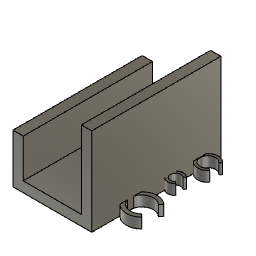
3dprentun v2 (Autodesk Fusion 360 design; units mm, degrees)
Autodesk Fusion 360 part; units mm, degrees
sketch "Sketch1" plane through (0, 0, 0) normal (0, 0, 1) x (1, 0, 0)
  line L0 (0, 0) -> (30.5, 0)
  line L1 (30.5, 0) -> (30.5, 50)
  line L2 (30.5, 50) -> (0, 50)
  line L3 (0, 50) -> (0, 0)
  dimension "d3" = 30.5
  dimension "d5" = 50
  constraint coincident L0.start L3.end
  constraint horizontal L0
  constraint perpendicular L0 L1
  constraint perpendicular L1 L2
  constraint perpendicular L0 L3
  measures "d3" distance of L0.start L0.end
  measures "d5" distance of L0.end L1.end
extrude "Extrude1" add sketch "Sketch1" along normal blind 19 makes body 1
sketch "Sketch2" plane through (0, 0, 19) normal (0, 0, 1) x (-1, 0, 0)
  line L0 (0, -50) -> (0, 0)
  line L1 (0, 0) -> (-30.5, 0)
  line L2 (-30.5, 0) -> (-30.5, -50)
  line L3 (-30.5, -50) -> (0, -50)
  line L4 (0, -50) -> (-4, -50)
  line L5 (-4, -50) -> (-26.5, -50)
  line L6 (-26.5, -50) -> (-26.5, 0)
  line L7 (-26.5, 0) -> (-4, 0)
  line L8 (-4, 0) -> (-4, -50)
  dimension "d9" = 4
  dimension "d10" = 22.5
  constraint coincident L0.start L3.end
  constraint coincident L3 L4.end
  constraint horizontal L5
  constraint vertical L6
  constraint horizontal L7
  constraint vertical L8
  constraint coincident L1 L6.end
  measures "d9" distance of L0.start L4.end
  measures "d10" distance of L6.end L7.end
extrude "Extrude2" cut sketch "Sketch2" against normal blind 15 contours L1 L3 L5 L6 L7 L8 bodies 1
sketch "Sketch3" plane through (0, 0, 4) normal (0, 0, 1) x (-1, 0, 0)
  line L0 (-4, 0) -> (-26.5, 0)
  line L1 (-26.5, 0) -> (-26.5, -50)
  line L2 (-26.5, -50) -> (-4, -50)
  line L3 (-4, -50) -> (-4, 0)
  circle A0 centre (-53.2527, -36.6298) radius 3
  circle A1 centre (-53.2527, -36.6298) radius 4
  dimension "d15" = 6
  dimension "d16" = 8
  constraint concentric A0 A1
  measures "d15" diameter of A0
  measures "d16" diameter of A1
extrude "Extrude3" add sketch "Sketch3" along normal blind 4 separate body contours A1 makes body 2
sketch "Sketch4" plane through (0, 0, 8) normal (0, 0, 1) x (-1, 0, 0)
  circle A0 centre (-53.2527, -36.6298) radius 3
  circle A1 centre (-53.2527, -36.6298) radius 4
  arc A2 (-56.3995, -34.1605) -> (-56.3725, -39.1331) centre (-53.2527, -36.6298) ccw
  line L0 (-56.3995, -34.1605) -> (-53.2527, -36.6298)
  line L1 (-53.2527, -36.6298) -> (-56.3725, -39.1331)
  constraint coincident A1 A2.end
  constraint coincident A0.centre A1.centre
extrude "Extrude4" cut sketch "Sketch4" against normal blind 4 contours A0 A1 A2 L0 L1 bodies 2
move_body "Move1" bodies 2 to x (1, 0, 0) y (0, 1, 0) z (0, 0, 1) at (-19.6373, -0.4364, 0)
move_body "Move2" bodies 2 to x (1, 0, 0) y (0, 1, 0) z (0, 0, 1) at (0, 5.6722, -3.8196)
combine "Combine1" operation add target body 2 tool bodies 1 keep tools
sketch "Sketch5" plane through (0, 0, 4) normal (0, 0, 1) x (-1, 0, 0)
  line L0 (-4, 0) -> (-26.5, 0)
  line L1 (-26.5, 0) -> (-26.5, -50)
  line L2 (-26.5, -50) -> (-4, -50)
  line L3 (-4, -50) -> (-4, 0)
  circle A0 centre (-41, -32) radius 2
  circle A1 centre (-41, -32) radius 3
  dimension "d21" = 4
  dimension "d22" = 6
  constraint concentric A0 A1
  measures "d21" diameter of A0
  measures "d22" diameter of A1
extrude "Extrude5" add sketch "Sketch5" along normal blind 4 separate body contours A1 makes body 3
sketch "Sketch6" plane through (0, 0, 8) normal (0, 0, 1) x (-1, 0, 0)
  circle A0 centre (-41, -32) radius 2
  circle A1 centre (-41, -32) radius 3
  arc A2 (-43.3273, -30.1069) -> (-42.8931, -34.3273) centre (-41, -32) ccw
  line L0 (-41, -32) -> (-43.3273, -30.1069) construction
  line L1 (-41, -32) -> (-42.8931, -34.3273) construction
  line L2 (-41, -32) -> (-42.8931, -34.3273)
  line L3 (-41, -32) -> (-43.3273, -30.1069)
  dimension "d25" = 90
  constraint coincident A1 A2.end
  constraint coincident A0.centre A1.centre
  measures "d25" angle of L0 L1
extrude "Extrude6" cut sketch "Sketch6" against normal blind 4 contours A0 A1 A2 L2 L3 bodies 3
move_body "Move3" bodies 3 to x (0.996195, -0.087156, 0) y (0.087156, 0.996195, 0) z (0, 0, 1) at (-2.633, 3.6952, 0)
move_body "Move4" bodies 3 to x (1, 0, 0) y (0, 1, 0) z (0, 0, 1) at (-8.6186, -1.091, 0)
move_body "Move5" bodies 3 to x (1, 0, 0) y (0, 1, 0) z (0, 0, 1) at (0, -0.3273, -3.9275)
sketch "Sketch7" plane through (0, 0, 4) normal (0, 0, 1) x (-1, 0, 0)
  line L0 (-4, 0) -> (-26.5, 0)
  line L1 (-26.5, 0) -> (-26.5, -50)
  line L2 (-26.5, -50) -> (-4, -50)
  line L3 (-4, -50) -> (-4, 0)
  circle A0 centre (-44, -24) radius 4.5
  circle A1 centre (-44, -24) radius 6
  dimension "d29" = 9
  dimension "d30" = 12
  constraint concentric A0 A1
  measures "d29" diameter of A0
  measures "d30" diameter of A1
extrude "Extrude7" add sketch "Sketch7" along normal blind 4 separate body contours A1 makes body 4
sketch "Sketch8" plane through (0, 0, 8) normal (0, 0, 1) x (-1, 0, 0)
  circle A0 centre (-44, -24) radius 4.5
  circle A1 centre (-44, -24) radius 6
  arc A2 (-48.5279, -20.0632) -> (-47.9368, -28.5279) centre (-44, -24) ccw
  line L0 (-44, -24) -> (-48.5279, -20.0632) construction
  line L1 (-44, -24) -> (-47.9368, -28.5279) construction
  line L2 (-44, -24) -> (-47.9368, -28.5279)
  line L3 (-44, -24) -> (-48.5279, -20.0632)
  dimension "d33" = 90
  constraint coincident A1 A2.end
  constraint coincident A0.centre A1.centre
  measures "d33" angle of L0 L1
extrude "Extrude8" cut sketch "Sketch8" against normal blind 4 contours A0 A1 A2 L2 L3 bodies 4
move_body "Move6" bodies 4 to x (1, 0, 0) y (0, 1, 0) z (0, 0, 1) at (-16.002, -9.23, -4.0366)
move_body "Move7" bodies 4 to x (0.997564, -0.069756, 0) y (0.069756, 0.997564, 0) z (0, 0, 1) at (-0.6765, 2.2953, 0)
move_body "Move8" bodies 4 to x (1, 0, 0) y (0, 1, 0) z (0, 0, 1) at (6.5458, 0, 0)
combine "Combine2" operation add target body 4 tool bodies 1 keep tools
extrude "Extrude9" add 1 faces at (27.8333, 33.3333, 19) along direction (0, 0, 1) blind 15 on bodies 1 bodies 1 3 2 4
equation "lengdborð = 22.5 mm"
equation "þykkt = 4 mm"
equation "d3 = þykkt * 2 + lengdborð"
equation "breidd = 50 mm"
equation "d5 = breidd"
equation "griplengd = 15 mm"
equation "d7 = griplengd + þykkt"
equation "d9 = þykkt"
equation "d10 = lengdborð"
equation "d11 = -griplengd"
equation "þvermálusbc = 6 mm"
equation "þvermállightning = 4 mm"
equation "d15 = þvermálusbc"
equation "d16 = þvermálusbc + 2 mm"
equation "d17 = þykkt"
equation "d19 = -þykkt"
equation "d21 = þvermállightning"
equation "d22 = þvermállightning + 2 mm"
equation "d23 = þykkt"
equation "d26 = -þykkt"
equation "þvermálhdmi = 9 mm"
equation "d29 = þvermálhdmi"
equation "d30 = þvermálhdmi + 3 mm"
equation "d31 = þykkt"
equation "d34 = -þykkt"
equation "d36 = griplengd"
